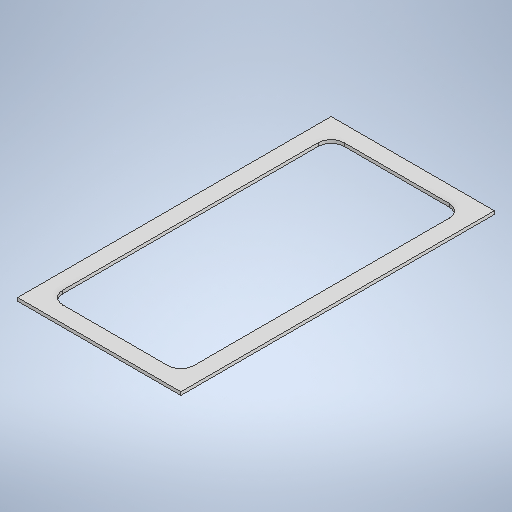
# Autodesk Inventor part: manija_puerta_marco_front_right
Saved by Autodesk Inventor 2025.1 (Build 291241020, 241B)
## iProperties
Created: 2024-12-04
Part Number: manija_puerta_marco_front_right
Material: Genérico
Document SubType Name: Modeling
Designer: ctamashiro
Density: 1 g/cm^3
Appearance: Valor por defecto
Author: ctamashiro
Autodesk Inventor part; units mm, degrees
ref_plane "YZ Plane" through (0, 0, 0) normal (1, 0, 0) x (0, 1, 0)
ref_plane "XZ Plane" through (0, 0, 0) normal (0, 1, 0) x (-1, 0, 0)
ref_plane "XY Plane" through (0, 0, 0) normal (0, 0, 1) x (1, 0, 0)
sketch "Boceto1" plane through (0, 0, 0) normal (0, 1, 0) x (-1, 0, 0)
  line L0 (20.25, -43.5) -> (-20.25, -43.5)
  line L1 (-20.25, -43.5) -> (-20.25, 43.5)
  line L2 (-20.25, 43.5) -> (20.25, 43.5)
  line L3 (20.25, 43.5) -> (20.25, -43.5)
  line L4 (20.25, -43.5) -> (-20.25, 43.5) construction
  line L5 (-20.25, -43.5) -> (20.25, 43.5) construction
  line L6 (25.25, -48.5) -> (-25.25, -48.5)
  line L7 (-25.25, -48.5) -> (-25.25, 48.5)
  line L8 (-25.25, 48.5) -> (25.25, 48.5)
  line L9 (25.25, 48.5) -> (25.25, -48.5)
  point P0 (0, 0)
  dimension "d0" = 40.5
  dimension "d1" = 87
  dimension "d2" = 5
  constraints: 20 end point, 4 parallel, 2 midpoint, 2 perpendicular, 1 horizontal, 3 other
  measures "d0" distance of L1.end L2.end
  measures "d1" distance of L0.end L1.end
  measures "d2" distance between parallel lines of L3 L9
extrude "Extrusión1" add sketch "Boceto1" along normal blind 1
fillet "Empalme1" radius 4 4 edges at (-20.25, 0.5, -43.5) (-20.25, 0.5, 43.5) (20.25, 0.5, -43.5) (20.25, 0.5, 43.5)
